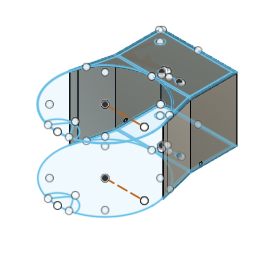
Engine Cap (Autodesk Fusion 360 design; units mm, degrees)
Autodesk Fusion 360 part; units mm, degrees
note: some values were not read from the file. Set by a fixed rule: which sketch regions a step uses.
sketch "Sketch1" plane through (0, 0, 0) normal (0, 0, 1) x (1, 0, 0)
  line L0 (-45, 112.5) -> (-43, 112.5)
  circle A0 centre (-32.1714, 98.7639) radius 4.5
  circle A1 centre (-33.5876, 33.5876) radius 2.15
  line L1 (-43, 110.5) -> (-43, 59.5)
  line L2 (-43, 59.5) -> (-43, 57.5)
  line L3 (-45, 57.5) -> (-55.8148, 13.8189)
  line L4 (-45, 112.5) -> (-45, 110.5)
  circle A2 centre (33.5876, -33.5876) radius 2.15
  line L5 (-43, 57.5) -> (-50.3698, 27.7333)
  line L6 (0, 0) -> (47.5, 0) construction
  circle A3 centre (33.5876, 33.5876) radius 2.15
  line L7 (2.9, 66.8243) -> (2.9, 70.1757)
  line L8 (18.1, 66.8243) -> (18.1, 70.1757)
  line L9 (0, 71.85) -> (2.9, 70.1757)
  line L10 (-2.9, 68.5) -> (-2.9, 66.8243)
  line L11 (0, 65.15) -> (2.9, 66.8243)
  line L12 (21, 71.85) -> (23.9, 70.1757)
  line L13 (2.9, 65.15) -> (3.3486, 65.15) construction
  line L14 (0, 68.5) -> (2.9, 68.5)
  circle A4 centre (0, 68.5) radius 2
  line L15 (2.9, 68.5) -> (-2.9, 68.5)
  line L16 (0, 68.5) -> (10.5, 68.5)
  line L17 (43, 57.5) -> (50.3698, 27.7333)
  line L18 (23.9, 68.5) -> (23.9, 66.8243)
  line L19 (45, 57.5) -> (45, 112.5)
  line L20 (0, 112.5) -> (45, 112.5)
  line L21 (-2.9, 66.8243) -> (-2.9, 70.1757)
  line L22 (0, 68.5) -> (21, 68.5)
  line L23 (45, 112.5) -> (-45, 112.5)
  line L24 (45, 57.5) -> (55.8148, 13.8189)
  line L25 (0, 57.5) -> (0, 64.5)
  line L26 (0, 71.85) -> (3.3486, 71.85) construction
  line L27 (0, 65.15) -> (3.3486, 65.15) construction
  line L28 (0, 68.5) -> (0, 65.15)
  line L29 (43, 59.5) -> (43, 57.5)
  line L30 (43, 59.5) -> (43, 110.5)
  line L31 (23.9, 66.8243) -> (23.9, 70.1757)
  line L32 (21, 65.15) -> (23.9, 66.8243)
  line L33 (10.5, 68.5) -> (10.5, 67) construction
  line L34 (0, 65.15) -> (0, 71.4)
  line L35 (0, 65.15) -> (-2.9, 66.8243)
  circle A5 centre (21, 68.5) radius 2
  line L36 (43, 110.5) -> (-43, 110.5)
  arc A6 (0, -38.75) -> (-18.4136, -54.4719) centre (0.0809, -57.4888) ccw
  spline S0 degree 2 poles (-12.8388, -56.0483) (0, -36) (12.5423, -56.1154) knots 0 0 0 4.029531 4.029531 4.029531 weights 1 3.529401 1
  line L37 (-43, 59.5) -> (43, 59.5)
  line L38 (0, 64.5) -> (0, 68.5)
  line L39 (43, 57.5) -> (-43, 57.5)
  line L40 (0, 0) -> (47.5, 0) construction
  line L41 (21, 71.85) -> (18.1, 70.1757)
  circle A7 centre (0, 0) radius 57.5
  line L42 (0, 0) -> (47.5, 0) construction
  line L43 (0, 0) -> (47.5, 0) construction
  line L44 (21, 65.15) -> (18.1, 66.8243)
  line L45 (2.9, 68.5) -> (2.9, 66.8243)
  arc A8 (18.5394, -54.4292) -> (0, -38.75) centre (0.0426, -57.5) ccw
  line L46 (2.9, 71.85) -> (2.9, 72.5)
  line L47 (0, 71.85) -> (-2.9, 70.1757)
  line L48 (-45, 57.5) -> (-45, 112.5)
  circle A9 centre (-33.5876, -33.5876) radius 2.15
  line L49 (-46, 112.5) -> (-46, 57.5)
  line L50 (-46, 57.5) -> (-56.81, 13.8189)
  line L51 (-46, 57.5) -> (-1.0012, 57.5) construction
  line L52 (-56.81, 13.8189) -> (-55.8148, 13.8189)
  line L53 (-46, 112.5) -> (-46, 113.5)
  line L54 (-46, 113.5) -> (46, 113.5)
  line L55 (46, 113.5) -> (46, 57.5)
  line L56 (46, 57.5) -> (56.8148, 13.8189)
  line L57 (56.8148, 13.8189) -> (55.8148, 13.8189)
  dimension "d1" = 115
  dimension "d26" = 4.3
  dimension "d27" = 4.3
  dimension "d28" = 4.3
  dimension "d29" = 4.3
  dimension "d8" = 18.75
  dimension "d63" = 90
  dimension "d64" = 55
  dimension "d65" = 2
  dimension "d66" = 2
  dimension "d67" = 51
  dimension "d68" = 86
  dimension "d69" = 2
  dimension "d76" = 7
  dimension "d77" = 4
  dimension "d78" = 21
  dimension "d79" = 4
  dimension "d80" = 4
  dimension "d81" = 3.35
  dimension "d82" = 6.7
  dimension "d83" = 2.9
  dimension "d84" = 5.8
  dimension "d85" = 150
  dimension "d86" = 30
  dimension "d87" = 30
  dimension "d88" = 60
  dimension "d89" = 10.5
  dimension "d33" = 103.9
  dimension "d34" = 92
  constraint coincident L6.start L40.start
  constraint horizontal L6
  constraint horizontal L40
  constraint horizontal L43
  constraint horizontal L42
  constraint coincident A6.end A7
  constraint coincident A8.start A7
  constraint perpendicular L19 L20
  constraint perpendicular L23 L48
  constraint perpendicular L4 L23
  constraint perpendicular L0 L48
  constraint perpendicular L1 L39
  constraint perpendicular L19 L37
  constraint perpendicular L30 L37
  constraint perpendicular L1 L36
  constraint perpendicular L29 L39
  constraint parallel L17 L24
  constraint perpendicular L2 L39
  constraint parallel L3 L5
  constraint midpoint L25.start L39
  constraint perpendicular L25 L37
  constraint perpendicular L37 L38
  constraint perpendicular L22 L38
  constraint coincident L14.start A4.centre
  constraint coincident L22.end A5.centre
  constraint coincident L11.start L38
  constraint parallel L28 L34
  constraint perpendicular L14 L38
  constraint perpendicular L15 L34
  constraint perpendicular L10 L15
  constraint perpendicular L15 L21
  constraint horizontal L27
  constraint horizontal L13
  constraint horizontal L26
  constraint coincident L46.start L26
  constraint coincident L13.start L27
  constraint perpendicular L16 L45
  constraint perpendicular L22 L33
  constraint symmetric L32.start L11.start L33
  constraint symmetric L12.start L9.start L33
  constraint symmetric L18.start L10.start L33
  constraint symmetric L18.end L10.end L33
  constraint symmetric L8.start L7.start L33
  constraint symmetric L7.end L8.end L33
  constraint symmetric L21.end L12.end L33
  constraint horizontal L51
  constraint horizontal L52
  constraint perpendicular L19 L54
  constraint perpendicular L54 L55
  constraint parallel L24 L56
  constraint parallel L54 L57
  measures "d1" diameter of A7
  measures "d26" diameter of A9
  measures "d27" diameter of A2
  measures "d28" diameter of A3
  measures "d29" diameter of A1
  measures "d8" radius of A8
  measures "d63" distance of L19.end L0.start
  measures "d64" distance of L3.start L0.start
  measures "d65" distance of L0.start L4.end
  measures "d66" distance of L0.start L0.end
  measures "d67" distance of L1.end L1.start
  measures "d68" distance of L1.end L29.start
  measures "d69" distance of L1.end L2.end
  measures "d76" distance of L25.end L25.start
  measures "d77" distance of L25.end L14.start
  measures "d78" distance of L14.start L22.end
  measures "d79" diameter of A4
  measures "d80" diameter of A5
  measures "d81" distance of L11.start L14.start
  measures "d82" distance of L9.start L11.start
  measures "d83" distance of L14.end L14.start
  measures "d84" distance of L14.end L10.start
  measures "d85" angle of L27 L35
  measures "d86" angle of L11 L13
  measures "d87" angle of L9 L26
  measures "d88" angle of L9 L47
  measures "d89" distance of L14.start L16.end
  measures "d33" angle of L50 L51
  measures "d34" distance of L53.end L54.end
ref_plane "WorkPlane1" through (0, 0, 77.259) normal (0, 0, 1) x (1, 0, 0)
sketch "Sketch2" plane through (0, 0, 77.259) normal (0, 0, 1) x (1, 0, 0)
  circle A0 centre (33.5876, -33.5876) radius 2.15
  line L0 (0, 0) -> (47.5, 0) construction
  circle A1 centre (33.5876, 33.5876) radius 2.15
  circle A2 centre (-33.5876, 33.5876) radius 2.15
  spline S0 degree 2 poles (-12.8388, -56.0483) (0, -36) (12.5423, -56.1154) knots 0 0 0 4.029531 4.029531 4.029531 weights 1 3.529401 1
  line L1 (0, 0) -> (47.5, 0) construction
  line L2 (43, 57.5) -> (-43, 57.5)
  line L3 (21, 71.85) -> (23.9, 70.1757)
  line L4 (-45, 112.5) -> (-43, 112.5)
  line L5 (0, 71.85) -> (3.3486, 71.85) construction
  line L6 (-46, 112.5) -> (-46, 113.5)
  line L7 (21, 71.85) -> (18.1, 70.1757)
  line L8 (0, 65.15) -> (3.3486, 65.15) construction
  line L9 (-43, 110.5) -> (-43, 59.5)
  line L10 (0, 68.5) -> (2.9, 68.5)
  line L11 (0, 68.5) -> (21, 68.5)
  line L12 (10.5, 68.5) -> (10.5, 67) construction
  line L13 (43, 110.5) -> (-43, 110.5)
  line L14 (45, 112.5) -> (-45, 112.5)
  line L15 (2.9, 66.8243) -> (2.9, 70.1757)
  line L16 (-43, 57.5) -> (-50.3698, 27.7333)
  line L17 (0, 112.5) -> (45, 112.5)
  circle A3 centre (0, 68.5) radius 2
  line L18 (-46, 113.5) -> (46, 113.5)
  line L19 (-45, 112.5) -> (-45, 110.5)
  line L20 (2.9, 68.5) -> (2.9, 66.8243)
  line L21 (-43, 59.5) -> (43, 59.5)
  line L22 (0, 65.15) -> (2.9, 66.8243)
  circle A4 centre (-32.1714, 98.7639) radius 4.5
  line L23 (0, 68.5) -> (10.5, 68.5)
  line L24 (2.9, 68.5) -> (-2.9, 68.5)
  line L25 (-43, 59.5) -> (-43, 57.5)
  line L26 (0, 68.5) -> (0, 65.15)
  line L27 (-2.9, 66.8243) -> (-2.9, 70.1757)
  line L28 (21, 65.15) -> (23.9, 66.8243)
  line L29 (2.9, 65.15) -> (3.3486, 65.15) construction
  line L30 (0, 71.85) -> (2.9, 70.1757)
  line L31 (23.9, 66.8243) -> (23.9, 70.1757)
  line L32 (23.9, 68.5) -> (23.9, 66.8243)
  line L33 (0, 65.15) -> (-2.9, 66.8243)
  line L34 (0, 57.5) -> (0, 64.5)
  line L35 (18.1, 66.8243) -> (18.1, 70.1757)
  circle A5 centre (21, 68.5) radius 2
  line L36 (43, 59.5) -> (43, 57.5)
  line L37 (-2.9, 68.5) -> (-2.9, 66.8243)
  line L38 (0, 71.85) -> (-2.9, 70.1757)
  line L39 (46, 57.5) -> (56.8148, 13.8189)
  line L40 (45, 57.5) -> (45, 112.5)
  line L41 (43, 57.5) -> (50.3698, 27.7333)
  line L42 (0, 65.15) -> (0, 71.4)
  line L43 (45, 57.5) -> (55.8148, 13.8189)
  line L44 (-46, 57.5) -> (-1.0012, 57.5) construction
  line L45 (-45, 57.5) -> (-45, 112.5)
  line L46 (-46, 112.5) -> (-46, 57.5)
  line L47 (43, 59.5) -> (43, 110.5)
  line L48 (-45, 57.5) -> (-55.8148, 13.8189)
  line L49 (21, 65.15) -> (18.1, 66.8243)
  line L50 (-46, 57.5) -> (-56.81, 13.8189)
  line L51 (46, 113.5) -> (46, 57.5)
  line L52 (0, 64.5) -> (0, 68.5)
  line L53 (2.9, 71.85) -> (2.9, 72.5)
  circle A6 centre (0, 0) radius 57.5
  line L54 (0, 0) -> (47.5, 0) construction
  circle A7 centre (-33.5876, -33.5876) radius 2.15
  line L55 (56.8148, 13.8189) -> (55.8148, 13.8189)
  line L56 (-56.81, 13.8189) -> (-55.8148, 13.8189)
  line L57 (0, 0) -> (47.5, 0) construction
  arc A8 (0, -38.75) -> (-18.4136, -54.4719) centre (0.0809, -57.4888) ccw
  arc A9 (18.5394, -54.4292) -> (0, -38.75) centre (0.0426, -57.5) ccw
  circle A10 centre (0, 0) radius 58
  dimension "d36" = 115
  dimension "d37" = 4.3
  dimension "d38" = 4.3
  dimension "d39" = 4.3
  dimension "d40" = 4.3
  dimension "d41" = 18.75
  dimension "d42" = 90
  dimension "d43" = 55
  dimension "d44" = 2
  dimension "d45" = 2
  dimension "d46" = 51
  dimension "d47" = 86
  dimension "d48" = 2
  dimension "d49" = 7
  dimension "d50" = 4
  dimension "d51" = 21
  dimension "d52" = 4
  dimension "d53" = 4
  dimension "d54" = 3.35
  dimension "d55" = 6.7
  dimension "d56" = 2.9
  dimension "d57" = 5.8
  dimension "d58" = 150
  dimension "d59" = 30
  dimension "d60" = 30
  dimension "d61" = 60
  dimension "d62" = 10.5
  dimension "d70" = 103.9
  dimension "d71" = 92
  dimension "d72" = 116
  constraint coincident L0.start L1.start
  constraint horizontal L57
  constraint horizontal L1
  constraint horizontal L0
  constraint horizontal L54
  constraint coincident A8.end A6
  constraint coincident A9.start A6
  constraint perpendicular L17 L40
  constraint perpendicular L14 L45
  constraint perpendicular L14 L19
  constraint perpendicular L4 L45
  constraint perpendicular L2 L9
  constraint perpendicular L21 L40
  constraint perpendicular L21 L47
  constraint perpendicular L9 L13
  constraint perpendicular L2 L36
  constraint parallel L41 L43
  constraint perpendicular L2 L25
  constraint parallel L16 L48
  constraint midpoint L34.start L2
  constraint perpendicular L21 L34
  constraint perpendicular L21 L52
  constraint perpendicular L11 L52
  constraint coincident L10.start L11.start
  constraint coincident L11.end A5.centre
  constraint coincident L8.start L52
  constraint parallel L26 L42
  constraint perpendicular L10 L52
  constraint perpendicular L24 L42
  constraint perpendicular L24 L37
  constraint perpendicular L24 L27
  constraint horizontal L8
  constraint horizontal L29
  constraint horizontal L5
  constraint coincident L53.start L5
  constraint coincident L29.start L8
  constraint perpendicular L20 L23
  constraint perpendicular L11 L12
  constraint symmetric L8.start L28.start L12
  constraint symmetric L3.start L5.start L12
  constraint symmetric L24.end L32.start L12
  constraint symmetric L27.start L28.end L12
  constraint symmetric L15.start L35.start L12
  constraint symmetric L7.end L15.end L12
  constraint symmetric L3.end L27.end L12
  constraint horizontal L44
  constraint horizontal L56
  constraint perpendicular L18 L40
  constraint perpendicular L18 L51
  constraint parallel L39 L43
  constraint parallel L18 L55
  measures "d36" diameter of A6
  measures "d37" diameter of A7
  measures "d38" diameter of A0
  measures "d39" diameter of A1
  measures "d40" diameter of A2
  measures "d41" radius of A9
  measures "d42" distance of L4.start L14.start
  measures "d43" distance of L4.start L45.start
  measures "d44" distance of L4.start L19.end
  measures "d45" distance of L4.start L4.end
  measures "d46" distance of L9.end L9.start
  measures "d47" distance of L21.end L9.end
  measures "d48" distance of L2.end L9.end
  measures "d49" distance of L34.end L34.start
  measures "d50" distance of L34.end L10.start
  measures "d51" distance of L10.start L11.end
  measures "d52" diameter of A3
  measures "d53" diameter of A5
  measures "d54" distance of L8.start L10.start
  measures "d55" distance of L8.start L5.start
  measures "d56" distance of L10.start L10.end
  measures "d57" distance of L10.end L24.end
  measures "d58" angle of L8 L33
  measures "d59" angle of L22 L29
  measures "d60" angle of L5 L30
  measures "d61" angle of L30 L38
  measures "d62" distance of L12.start L10.start
  measures "d70" angle of L44 L50
  measures "d71" distance of L6.end L18.end
  measures "d72" diameter of A10
extrude "Extrude2" add sketch "Sketch2" against normal blind 1 contours L4 L6 L14 L17 L18 L19 L39 L40 L43 L45 L46 L48 L50 L51 L55 L56 A10 | L4 L9 L13 L14 L16 L17 L19 L25 L36 L40 L41 L43 L45 L47 L48 A10 | L2 L16 A10 | L2 L21 L25 L34 A10 | L2 L21 L34 L36 A10 | L2 L41 A10 | L9 L13 L21 L47 | L3 L7 L28 L31 L32 L35 L49 | L10 L11 A3 L23 L24 L42 | A3 L24 L26 L42 L52 | L10 L11 A3 L23 L24 L26 L42 L52 | A3 L24 L42 | L10 L11 L15 A3 L23 L24 L27 L30 L38 | L10 L11 L15 A3 L20 L22 L23 L24 L26 L42 L52 | A3 L24 L26 L27 L33 L37 L42 L52 | A4 | A5 makes body 1
extrude "Extrude1" add sketch "Sketch2" against normal blind 77.256 separate body contours L4 L6 L14 L17 L18 L19 L39 L40 L43 L45 L46 L48 L50 L51 L55 L56 A10 makes body 2
sketch "Sketch3" plane through (46, 0, 0) normal (1, 0, 0) x (0, 1, 0)
  line L0 (113.5, 77.259) -> (57.5, 77.259)
  line L1 (57.5, 77.259) -> (57.5, 0.003)
  line L2 (57.5, 0.003) -> (113.5, 0.003)
  line L3 (113.5, 0.003) -> (113.5, 77.259)
  line L4 (57.5, 0.003) -> (70, 0.003)
  line L5 (70, 0.003) -> (70, 3.003)
  circle A0 centre (70, 3.003) radius 2
  dimension "d91" = 12.5
  dimension "d92" = 3
  dimension "d93" = 4
  constraint coincident L1.end L2.start
  constraint coincident L2 L4.end
  constraint perpendicular L4 L5
  constraint coincident L5.end A0.centre
  measures "d91" distance of L1.end L4.end
  measures "d92" distance of L4.end L5.end
  measures "d93" diameter of A0
extrude "Extrude3" cut sketch "Sketch3" against normal blind 14 contours A0 bodies 2
sketch "Sketch4" plane through (-46, 0, 0) normal (-1, 0, 0) x (0, -1, 0)
  line L0 (-57.5, 77.259) -> (-113.5, 77.259)
  line L1 (-113.5, 77.259) -> (-113.5, 0.003)
  line L2 (-113.5, 0.003) -> (-57.5, 0.003)
  line L3 (-57.5, 0.003) -> (-57.5, 77.259)
  line L4 (-57.5, 0.003) -> (-70, 0.003)
  line L5 (-70, 0.003) -> (-70, 3.003)
  circle A0 centre (-70, 3.003) radius 2
  dimension "d96" = 12.5
  dimension "d97" = 3
  dimension "d98" = 4
  constraint coincident L2.end L3.start
  constraint coincident L2 L4.end
  constraint perpendicular L4 L5
  constraint coincident L5.end A0.centre
  measures "d96" distance of L2.end L4.end
  measures "d97" distance of L4.end L5.end
  measures "d98" diameter of A0
extrude "Extrude4" cut sketch "Sketch4" against normal blind 1 contours A0 bodies 2
sketch "Sketch5" plane through (0, 113.5, 0) normal (0, 1, 0) x (-1, 0, 0)
  line L0 (46, 77.259) -> (-46, 77.259)
  line L1 (-46, 77.259) -> (-46, 0.003)
  line L2 (-46, 0.003) -> (46, 0.003)
  line L3 (46, 0.003) -> (46, 77.259)
  line L4 (0, 0) -> (0, 3)
  circle A0 centre (0, 3) radius 2
  dimension "d101" = 3
  dimension "d102" = 4
  constraint coincident L4.start origin
  constraint perpendicular L2 L4
  constraint coincident L4.end A0.centre
  measures "d101" distance of L4.start L4.end
  measures "d102" diameter of A0
extrude "Extrude5" cut sketch "Sketch5" against normal blind 1 contours A0 bodies 2
equation "d8 = 17.250 mm + 1.5 mm"
equation "d67 = 53 mm - 2 mm"
equation "d68 = 88 mm - 2 mm"
equation "d81 = ( 6.7 / 2 ) * 1 mm"
equation "d83 = ( 5.8 / 2 ) * 1 mm"
equation "d89 = ( 21 / 2 ) * 1 mm"
equation "d33 = 90 deg + 13.9 deg"
equation "d35 = 71.259 mm + 6 mm"
equation "d41 = 17.250 mm + 1.5 mm"
equation "d46 = 53 mm - 2 mm"
equation "d47 = 88 mm - 2 mm"
equation "d54 = ( 6.7 / 2 ) * 1 mm"
equation "d56 = ( 5.8 / 2 ) * 1 mm"
equation "d62 = ( 21 / 2 ) * 1 mm"
equation "d70 = 90 deg + 13.9 deg"
equation "d73 = -71.256 mm + -6 mm"
